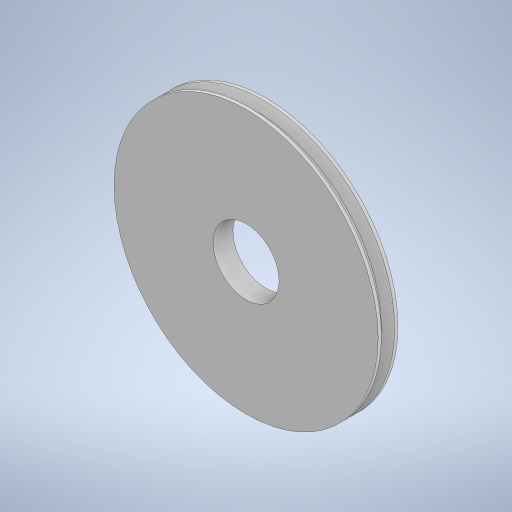
# Autodesk Inventor part: kladicka
Saved by Autodesk Inventor 2023.1 (Build 271208000, 208)
## iProperties
Created: 2023-11-22
Part Number: kladicka
Material: Generic
Document SubType Name: Modeling
Designer: zavrel
Density: 1 g/cm^3
Appearance: Default
Author: zavrel
Autodesk Inventor part; units mm, degrees
ref_plane "YZ Plane" through (0, 0, 0) normal (1, 0, 0) x (0, 1, 0)
ref_plane "XZ Plane" through (0, 0, 0) normal (0, 1, 0) x (-1, 0, 0)
ref_plane "XY Plane" through (0, 0, 0) normal (0, 0, 1) x (1, 0, 0)
sketch "Sketch1" plane through (0, 0, 0) normal (0, 1, 0) x (-1, 0, 0)
  line L0 (9.5, 0.1897) -> (10, 0.6897)
  line L1 (10, 0.6897) -> (10, 0.9397)
  line L2 (10, 0.9397) -> (0, 0.9397)
  line L3 (9.5, 0.1897) -> (-0.1607, 0.1897) construction
  line L4 (9.5, 0.1897) -> (10, -0.3103)
  line L5 (10, -0.3103) -> (10, -0.5603)
  line L6 (10, -0.5603) -> (0, -0.5603)
  line L7 (0, 0.9397) -> (0, -0.5603)
  dimension "d1" = 1.5
  dimension "d2" = 1
  dimension "d3" = 90
  constraints: 16 end point, 3 symmetric about line, 2 vertical, 1 horizontal, 1 perpendicular
  measures "d1" distance between parallel lines of L2 L6
  measures "d2" distance of L4.end L0.end
  measures "d3" angle of L4 L0
revolve "Revolution1" add sketch "Sketch1" angle 360 about axis through (0, 0, 0.9397) along (0, 0, -1)
sketch "Sketch2" plane through (0, 0, -0.5603) normal (0, 0, -1) x (-1, 0, 0)
  circle A0 centre (0, 0) radius 10 projected
  circle A1 centre (0, 0) radius 2.5
  point P0 (0, 0)
  dimension "d5" = 5
  constraints: 1 centre point, 1 coincident
  measures "d5" diameter of A1
extrude "Extrusion1" cut sketch "Sketch2" against normal blind 10 contours A1
body "Solid1"
